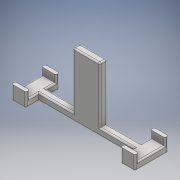
# Autodesk Inventor part: handle2
Saved by Autodesk Inventor 2016 (Build 200138000, 138)
## iProperties
Created: 2016-05-24
Part Number: handle2
Material: ABS Plastic
Document SubType Name: Modeling
Designer: Hamid Osooli
Density: 1.06 g/cm^3
Appearance: Smooth - White
Mass: 34.3484 g
Surface Area: 120.272 cm^2
Volume: 32.4042 cm^3
Author: Hamid Osooli
Autodesk Inventor part; units mm, degrees
ref_plane "YZ Plane" through (0, 0, 0) normal (1, 0, 0) x (0, 1, 0)
ref_plane "XZ Plane" through (0, 0, 0) normal (0, 1, 0) x (-1, 0, 0)
ref_plane "XY Plane" through (0, 0, 0) normal (0, 0, 1) x (1, 0, 0)
sketch "Sketch1" plane through (0, 0, 0) normal (0, 0, 1) x (1, 0, 0)
  line L0 (-82.75, 18) -> (-67.25, 18)
  line L1 (-65.25, 20) -> (-65.25, 21)
  line L2 (-67.25, 23) -> (-82.75, 23)
  line L3 (-84.75, 21) -> (-84.75, 20)
  line L4 (-82.75, -23) -> (-67.25, -23)
  line L5 (-65.25, -21) -> (-65.25, -20)
  line L6 (-67.25, -18) -> (-82.75, -18)
  line L7 (-84.75, -20) -> (-84.75, -21)
  line L8 (67.25, 18) -> (82.75, 18)
  line L9 (84.75, 20) -> (84.75, 21)
  line L10 (82.75, 23) -> (67.25, 23)
  line L11 (65.25, 21) -> (65.25, 20)
  line L12 (67.25, -23) -> (82.75, -23)
  line L13 (84.75, -21) -> (84.75, -20)
  line L14 (82.75, -18) -> (67.25, -18)
  line L15 (65.25, -20) -> (65.25, -21)
  arc A0 (-65.25, 21) -> (-67.25, 23) centre (-67.25, 21) ccw
  arc A1 (-67.25, 18) -> (-65.25, 20) centre (-67.25, 20) ccw
  arc A2 (-84.75, 20) -> (-82.75, 18) centre (-82.75, 20) ccw
  arc A3 (-82.75, 23) -> (-84.75, 21) centre (-82.75, 21) ccw
  arc A4 (-82.75, -18) -> (-84.75, -20) centre (-82.75, -20) ccw
  arc A5 (-65.25, -20) -> (-67.25, -18) centre (-67.25, -20) ccw
  arc A6 (-67.25, -23) -> (-65.25, -21) centre (-67.25, -21) ccw
  arc A7 (-84.75, -21) -> (-82.75, -23) centre (-82.75, -21) ccw
  arc A8 (67.25, 23) -> (65.25, 21) centre (67.25, 21) ccw
  arc A9 (84.75, 21) -> (82.75, 23) centre (82.75, 21) ccw
  arc A10 (65.25, 20) -> (67.25, 18) centre (67.25, 20) ccw
  arc A11 (82.75, 18) -> (84.75, 20) centre (82.75, 20) ccw
  arc A12 (84.75, -20) -> (82.75, -18) centre (82.75, -20) ccw
  arc A13 (82.75, -23) -> (84.75, -21) centre (82.75, -21) ccw
  arc A14 (65.25, -21) -> (67.25, -23) centre (67.25, -21) ccw
  arc A15 (67.25, -18) -> (65.25, -20) centre (67.25, -20) ccw
  line L16 (-35, 23) -> (35, 23)
  line L17 (35, -23) -> (-35, -23)
  point P0 (-65.25, 23)
  point P1 (-65.25, 18)
  point P2 (-84.75, 23)
  point P3 (-65.25, -18)
  point P4 (-65.25, -23)
  point P5 (-84.75, -18)
  point P6 (84.75, 23)
  point P7 (84.75, 18)
  point P8 (65.25, 23)
  point P9 (65.25, -23)
  point P10 (84.75, -18)
  point P11 (84.75, -23)
  point P12 (65.25, -18)
  dimension "d22" = 19.5
  dimension "d23" = 5
  dimension "d24" = 19.5
  dimension "d25" = 5
  dimension "d26" = 19.5
  dimension "d27" = 5
  dimension "d28" = 19.5
  dimension "d29" = 5
  dimension "d30" = 2
  dimension "d85" = 70
  constraints: 36 end point, 32 point on circle, 32 tangent, 27 point on line, 16 centre point, 15 equal radius, 8 parallel, 4 horizontal, 4 perpendicular
  measures "d22" distance of point (-84.75, 23) point (-65.25, 23)
  measures "d23" distance of point (-65.25, 23) point (-65.25, 18)
  measures "d24" distance of point (-84.75, -18) point (-65.25, -18)
  measures "d25" distance of point (-65.25, -18) point (-65.25, -23)
  measures "d26" distance of point (65.25, 23) point (84.75, 23)
  measures "d27" distance of point (84.75, 23) point (84.75, 18)
  measures "d28" distance of point (65.25, -18) point (84.75, -18)
  measures "d29" distance of point (84.75, -18) point (84.75, -23)
  measures "d30" radius of A0
  measures "d85" distance of L16.start L16.end
extrude "Extrusion1" add sketch "Sketch1" along normal blind 10
sketch "Sketch2" plane through (0, 0, 0) normal (0, 0, 1) x (1, 0, 0)
  line L0 (67.25, -23) -> (82.75, -23)
  line L1 (84.75, -21) -> (84.75, 21)
  line L2 (82.75, 23) -> (67.25, 23)
  line L3 (65.25, 21) -> (65.25, -21)
  line L4 (-82.75, -23) -> (-67.25, -23)
  line L5 (-65.25, -21) -> (-65.25, 21)
  line L6 (-67.25, 23) -> (-82.75, 23)
  line L7 (-84.75, 21) -> (-84.75, -21)
  arc A0 (-65.25, 21) -> (-67.25, 23) centre (-67.25, 21) ccw
  arc A1 (-82.75, 23) -> (-84.75, 21) centre (-82.75, 21) ccw
  arc A2 (-67.25, -23) -> (-65.25, -21) centre (-67.25, -21) ccw
  arc A3 (-84.75, -21) -> (-82.75, -23) centre (-82.75, -21) ccw
  arc A4 (65.25, -21) -> (67.25, -23) centre (67.25, -21) ccw
  arc A5 (82.75, -23) -> (84.75, -21) centre (82.75, -21) ccw
  arc A6 (84.75, 21) -> (82.75, 23) centre (82.75, 21) ccw
  arc A7 (67.25, 23) -> (65.25, 21) centre (67.25, 21) ccw
  point P0 (0, 0)
  point P1 (84.75, 23)
  point P2 (84.75, -23)
  point P3 (65.25, 23)
  point P4 (-65.25, 23)
  point P5 (-65.25, -23)
  point P6 (-84.75, 23)
  dimension "d32" = 19.5
  dimension "d33" = 46
  dimension "d34" = 19.5
  dimension "d35" = 46
  dimension "d36" = 2
  constraints: 16 end point, 16 point on circle, 16 tangent, 12 point on line, 8 centre point, 7 equal radius, 4 parallel, 2 horizontal, 2 perpendicular
  measures "d32" distance of point (65.25, 23) point (84.75, 23)
  measures "d33" distance of point (84.75, 23) point (84.75, -23)
  measures "d34" distance of point (-84.75, 23) point (-65.25, 23)
  measures "d35" distance of point (-65.25, 23) point (-65.25, -23)
  measures "d36" radius of A0
extrude "Extrusion2" add sketch "Sketch2" against normal blind 10
sketch "Sketch4" plane through (65.25, -20, 0) normal (-1, 0, 0) x (0, 0, 1)
  line L0 (0, 40) -> (0, 0) projected
  line L1 (-10, 41) -> (-10, -1) projected
  line L2 (0, 15) -> (-10, 15)
  line L3 (-10, 15) -> (-10, 25)
  line L4 (-10, 25) -> (0, 25)
  line L5 (0, 25) -> (0, 15)
  point P0 (0, 20)
  dimension "d37" = 10
  constraints: 8 end point, 2 parallel, 2 point on line, 1 horizontal, 1 perpendicular
  measures "d37" distance of L2.end L3.end
extrude "Extrusion4" add sketch "Sketch4" along normal up to next
sketch "Sketch5" plane through (0, 0, 0) normal (0, 0, 1) x (1, 0, 0)
  line L0 (65.25, -5) -> (-65.25, -5) projected
  line L1 (65.25, 5) -> (-65.25, 5) projected
  line L2 (-18.5, -5) -> (18.5, -5)
  line L3 (18.5, -5) -> (18.5, 5)
  line L4 (18.5, 5) -> (-18.5, 5)
  line L5 (-18.5, 5) -> (-18.5, -5)
  dimension "d41" = 37
  constraints: 8 end point, 2 parallel, 2 point on line, 1 horizontal, 1 perpendicular
  measures "d41" distance of L4.end L3.end
extrude "Extrusion5" add sketch "Sketch5" along normal blind 77
sketch "Sketch6" plane through (65.25, 5, 0) normal (0, 1, 0) x (1, 0, 0)
  line L0 (-77, -5) -> (-53.5, -5)
  line L1 (-51.5, -7) -> (-51.5, -70)
  line L2 (-53.5, -72) -> (-77, -72)
  line L3 (-79, -70) -> (-79, -7)
  arc A0 (-51.5, -7) -> (-53.5, -5) centre (-53.5, -7) ccw
  arc A1 (-79, -70) -> (-77, -72) centre (-77, -70) ccw
  arc A2 (-53.5, -72) -> (-51.5, -70) centre (-53.5, -70) ccw
  arc A3 (-77, -5) -> (-79, -7) centre (-77, -7) ccw
  point P0 (-65.25, 0)
  point P1 (-51.5, -72)
  point P2 (-51.5, -5)
  point P3 (-79, -72)
  dimension "d44" = 27.5
  dimension "d45" = 67
  dimension "d63" = 2
  dimension "d64" = 2
  constraints: 8 end point, 8 point on circle, 8 tangent, 6 point on line, 4 centre point, 2 equal radius, 2 parallel, 1 horizontal, 1 perpendicular
  measures "d44" distance of point (-51.5, -72) point (-79, -72)
  measures "d45" distance of point (-51.5, -5) point (-51.5, -72)
  measures "d63" radius of A0
  measures "d64" radius of A1
extrude "Extrusion6" cut sketch "Sketch6" against normal blind 5
sketch "Sketch7" plane through (65.25, 0, 0) normal (0, 1, 0) x (1, 0, 0)
  circle A0 centre (-74.25, -8.5) radius 1.75
  circle A1 centre (-56.25, -8.5) radius 1.75
  circle A2 centre (-56.25, -68.5) radius 1.75
  circle A3 centre (-74.25, -68.5) radius 1.75
  point P0 (-65.25, 0)
  dimension "d73" = 3.5
  dimension "d74" = 3.5
  dimension "d75" = 3.5
  dimension "d76" = 3.5
  constraints: 4 centre point
  measures "d73" diameter of A0
  measures "d74" diameter of A1
  measures "d75" diameter of A2
  measures "d76" diameter of A3
extrude "Extrusion7" add sketch "Sketch7" along normal blind 5
fillet "Fillet1" radius 2 8 edges at (18.5, 5, 38.5) (-18.5, 5, 38.5) (0, 5, 77) (0, -5, 77) (18.5, 0, 77) (-18.5, 0, 77) (18.5, -5, 38.5) (-18.5, -5, 38.5)
fillet "Fillet2" radius 2 32 edges at (-65.25, 12.5, 0) (-65.25, -12.5, 0) (-84.75, 0, 0) (65.25, -12.5, 0) (65.25, 12.5, 0) (84.75, 0, 0) (84.1642, -22.4142, -10) (75, -23, -10) (65.8358, -22.4142, -10) (65.25, -13, -10) (84.1642, 22.4142, -10) (75, 23, -10) (65.8358, 22.4142, -10) (65.25, 13, -10) (84.75, 0, -10) (-65.8358, 22.4142, -10) (-75, 23, -10) (-84.1642, 22.4142, -10) (-84.75, 0, -10) (-84.1642, -22.4142, -10) (-75, -23, -10) (-65.8358, -22.4142, -10) (-65.25, -13, -10) (-65.25, 13, -10) (-17.5, 5, 0) (-41.875, 5, 0) (-17.5, -5, 0) (17.5, 5, 0) (41.875, 5, 0) (17.5, -5, 0) (0, 5, -10) (0, -5, -10)
sketch "Sketch8" plane through (-16.5, 5, 75) normal (0, 1, 0) x (1, 0, 0)
  line L0 (4.75, 70) -> (28.25, 70) projected
  line L1 (-50.75, 85) -> (83.75, 85) projected
  line L2 (11.5, 70) -> (21.5, 70)
  line L3 (21.5, 70) -> (21.5, 85)
  line L4 (21.5, 85) -> (11.5, 85)
  line L5 (11.5, 85) -> (11.5, 70)
  point P0 (16.5, 75)
  dimension "d81" = 10
  constraints: 8 end point, 2 parallel, 2 point on line, 1 horizontal, 1 perpendicular
  measures "d81" distance of L4.end L3.end
extrude "Extrusion8" cut sketch "Sketch8" against normal blind 5
fillet "Fillet3" radius 2 9 edges at (-5, 4.4142, -9.4142) (-5, 1.5, -10) (-5, 5, -1.5) (5, 4.4142, -9.4142) (5, 1.5, -10) (5, 5, -1.5) (-5, 2.5, 5) (5, 2.5, 5) (0, 0, -10)
body "Solid1"
